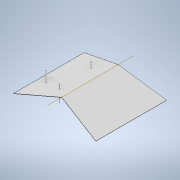
# Autodesk Inventor part: houseDormerRoof
Saved by Autodesk Inventor 2022.1 (Build 261234000, 234)
## iProperties
Created: 2021-07-13
Part Number: houseDormerRoof
Material: Generic
Document SubType Name: Modeling
Designer: robst
Density: 1 g/cm^3
Appearance: Default
Author: robst
Autodesk Inventor part; units mm, degrees
ref_plane "YZ Plane" through (0, 0, 0) normal (1, 0, 0) x (0, 1, 0)
ref_plane "Work Plane3" through (0, 0, 0) normal (-0.3162278, 0.9486833, 0) x (0, 0, 1)
sketch "Sketch5" plane through (0, 0, 0) normal (-0.3162278, 0.9486833, 0) x (0, 0, 1)
  line L0 (0, 0) -> (-5486.4, 0)
  line L1 (-5486.4, 0) -> (-6172.2, -4216.4)
  line L2 (-6172.2, -4216.4) -> (685.8, -4216.4)
  line L3 (685.8, -4216.4) -> (0, 0)
  line L4 (-7543.8, 0) -> (2057.4, 0) projected
  dimension "d14" = 5486.4
  dimension "d15" = 4216.4
  dimension "d18" = 6858
  constraints: 8 end point, 2 horizontal, 1 equal length, 1 parallel
  measures "d14" distance of L0.start L0.end
  measures "d15" distance between parallel lines of L0 L2
  measures "d18" distance of L1.end L2.end
ref_plane "Work Plane4" through (0, 0, 0) normal (0.3162278, 0.9486833, 0) x (0, 0, 1)
sketch "Sketch6" plane through (0, 0, 0) normal (0.3162278, 0.9486833, 0) x (0, 0, 1)
  line L0 (0, 0) -> (-5486.4, 0)
  line L1 (-5486.4, 0) -> (-6172.2, 4216.4)
  line L2 (-6172.2, 4216.4) -> (685.8, 4216.4)
  line L3 (685.8, 4216.4) -> (0, 0)
  dimension "d20" = 5486.4
  dimension "d21" = 6858
  dimension "d22" = 4216.4
  constraints: 8 end point, 1 equal length, 1 horizontal, 1 parallel
  measures "d20" distance of L0.start L0.end
  measures "d21" distance of L1.end L2.end
  measures "d22" distance between parallel lines of L2 L0
extrude "Extrusion3" add sketch "Sketch5" against normal blind 25.4
extrude "Extrusion4" add sketch "Sketch6" against normal blind 25.4
sketch "Sketch7" plane through (0, 0, 0) normal (0, 1, 0) x (-1, 0, 0)
  circle A0 centre (1555.0127, -4394.2578) radius 25.4
  circle A1 centre (1206.3632, -1004.6095) radius 25.4
  circle A2 centre (3007.7191, -1469.4756) radius 25.4
  point P0 (0, 0)
  dimension "d27" = 50.8
  constraints: 3 centre point, 2 equal radius
  measures "d27" diameter of A0
extrude "Extrusion5" add sketch "Sketch7" against normal blind 1524
equation "\"d14\" = dormerRidgeLineLength"
equation "\"d15\" = dormerRidgeToGarageEave"
equation "\"d18\" = dormerGarageEaveLength"
equation "\"d20\" = dormerRidgeLineLength"
equation "\"d21\" = dormerPoolEaveLength"
equation "\"d22\" = dormerRidgeToPoolEave"
equation "\"pitch_6_12\" = 26.565deg"
equation "\"d11\" = pitch_4_12"
equation "\"pitch_4_12\" = 18.434949deg"
equation "\"dormerRidgeLineLength\" = 5486.4"
equation "\"dormerPoolEaveLength\" = 6858"
equation "\"dormerGarageEaveLength\" = 6858"
equation "\"dormerRidgeToGarageEave\" = 4216.4"
equation "\"d19\" = -pitch_4_12"
equation "\"dormerRidgeToPoolEave\" = 4216.4"
body "Solid2"
